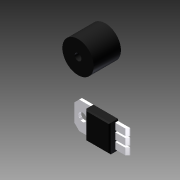
# Autodesk Inventor part: Breadboard
Saved by Autodesk Inventor 2012 (Build 160160000, 160)
## iProperties
Created: 2012-03-02
Part Number: Breadboard
Material: Default
Document SubType Name: Modeling
Designer: Lauszus
Density: 1 g/cm^3
Author: Lauszus
Autodesk Inventor part; units mm, degrees
ref_plane "YZ Plane" through (0, 0, 0) normal (1, 0, 0) x (0, 1, 0)
ref_plane "XZ Plane" through (0, 0, 0) normal (0, 1, 0) x (-1, 0, 0)
ref_plane "XY Plane" through (0, 0, 0) normal (0, 0, 1) x (1, 0, 0)
sketch "Sketch1" plane through (0, 0, 0) normal (0, 0, 1) x (1, 0, 0)
  line L0 (35.093, -7.2202) -> (-19.907, -7.2202)
  line L1 (-19.907, -7.2202) -> (-19.907, 74.7798)
  line L2 (-19.907, 74.7798) -> (35.093, 74.7798)
  line L3 (35.093, 74.7798) -> (35.093, -7.2202)
  line L4 (-1.6316, 73.7798) -> (15.8684, 73.7798)
  line L5 (15.8684, 73.7798) -> (15.8684, 38.2798)
  line L6 (15.8684, 38.2798) -> (-1.6316, 38.2798)
  line L7 (-1.6316, 38.2798) -> (-1.6316, 73.7798)
  circle A0 centre (7.5885, 28.2798) radius 5.75
  line L8 (12.233, 6.0025) -> (3.233, 6.0025)
  line L9 (3.233, 6.0025) -> (3.233, -3.9975)
  line L10 (3.233, -3.9975) -> (12.233, -3.9975)
  line L11 (12.233, -3.9975) -> (12.233, 6.0025)
  circle A1 centre (7.5885, 28.2798) radius 1.25
  line L12 (3.233, 6.0025) -> (-2.767, 6.0025)
  line L13 (-2.767, 6.0025) -> (-2.767, -3.9975)
  line L14 (-2.767, -3.9975) -> (3.233, -3.9975)
  line L15 (3.233, -3.9975) -> (3.233, 6.0025)
  line L16 (12.233, 5.3167) -> (16.7288, 5.3167)
  line L17 (16.7288, 5.3167) -> (16.7288, 2.7767)
  line L18 (16.7288, 2.7767) -> (12.233, 2.7767)
  line L19 (12.233, 2.7767) -> (12.233, 5.3167)
  line L20 (12.233, -1.5375) -> (12.233, 1.0025)
  line L21 (12.233, -3.4895) -> (12.233, -0.9495)
  line L22 (12.233, 2.2687) -> (16.7288, 2.2687)
  line L23 (16.7288, 2.2687) -> (16.7288, -0.2713)
  line L24 (16.7288, -0.2713) -> (12.233, -0.2713)
  line L25 (12.233, -0.2713) -> (12.233, 2.2687)
  line L26 (12.233, -0.7793) -> (16.7288, -0.7793)
  line L27 (16.7288, -0.7793) -> (16.7288, -3.3193)
  line L28 (16.7288, -3.3193) -> (12.233, -3.3193)
  line L29 (12.233, -3.3193) -> (12.233, -0.7793)
  circle A2 centre (0.233, 0.9987) radius 1.5
  circle A3 centre (0.3684, 66.2798) radius 0.75
  circle A4 centre (0.3684, 63.7398) radius 0.75
  circle A5 centre (0.3684, 61.1998) radius 0.75
  circle A6 centre (0.3684, 58.6598) radius 0.75
  circle A7 centre (0.3684, 56.1198) radius 0.75
  circle A8 centre (0.3684, 53.5798) radius 0.75
  circle A9 centre (0.3684, 51.0398) radius 0.75
  circle A10 centre (0.3684, 48.4998) radius 0.75
  circle A11 centre (13.8684, 66.2798) radius 0.75
  circle A12 centre (13.8684, 63.7398) radius 0.75
  circle A13 centre (13.8684, 61.1998) radius 0.75
  circle A14 centre (13.8684, 58.6598) radius 0.75
  circle A15 centre (13.8684, 56.1198) radius 0.75
  circle A16 centre (13.8684, 53.5798) radius 0.75
  circle A17 centre (13.8684, 51.0398) radius 0.75
  circle A18 centre (13.8684, 48.4998) radius 0.75
  line L30 (-17.907, 69.7798) -> (-16.407, 69.7798)
  line L31 (-16.407, 69.7798) -> (-16.407, -2.2202)
  line L32 (-16.407, -2.2202) -> (-17.907, -2.2202)
  line L33 (-17.907, -2.2202) -> (-17.907, 69.7798)
  line L34 (-15.367, -2.2202) -> (-13.867, -2.2202)
  line L35 (-13.867, -2.2202) -> (-13.867, 69.7798)
  line L36 (-13.867, 69.7798) -> (-15.367, 69.7798)
  line L37 (-15.367, 69.7798) -> (-15.367, -2.2202)
  line L38 (31.593, 69.7798) -> (33.093, 69.7798)
  line L39 (33.093, 69.7798) -> (33.093, -2.2202)
  line L40 (33.093, -2.2202) -> (31.593, -2.2202)
  line L41 (31.593, -2.2202) -> (31.593, 69.7798)
  line L42 (30.553, -2.2202) -> (29.053, -2.2202)
  line L43 (29.053, -2.2202) -> (29.053, 69.7798)
  line L44 (29.053, 69.7798) -> (30.553, 69.7798)
  line L45 (30.553, 69.7798) -> (30.553, -2.2202)
  line L46 (5.8684, 68.7798) -> (10.8684, 68.7798)
  line L47 (10.8684, 68.7798) -> (10.8684, 63.7798)
  line L48 (10.8684, 63.7798) -> (5.8684, 63.7798)
  line L49 (5.8684, 63.7798) -> (5.8684, 68.7798)
  line L50 (6.8684, 55.8198) -> (10.8684, 55.8198)
  line L51 (10.8684, 55.8198) -> (10.8684, 53.2798)
  line L52 (10.8684, 53.2798) -> (6.8684, 53.2798)
  line L53 (6.8684, 53.2798) -> (6.8684, 55.8198)
  line L54 (5.8684, 48.2798) -> (10.8684, 48.2798)
  line L55 (10.8684, 48.2798) -> (10.8684, 43.2798)
  line L56 (10.8684, 43.2798) -> (5.8684, 43.2798)
  line L57 (5.8684, 43.2798) -> (5.8684, 48.2798)
  circle A19 centre (0.8684, 71.2798) radius 1.5
  circle A20 centre (0.8684, 40.7798) radius 1.5
  point P0 (0, 0)
  dimension "d0" = 82
  dimension "d1" = 55
  dimension "d2" = 17.5
  dimension "d3" = 35.5
  dimension "d4" = 11.5
  dimension "d5" = 2.5
  dimension "d6" = 1
  dimension "d7" = 10
  dimension "d8" = 27.4955
  dimension "d9" = 9
  dimension "d10" = 10
  dimension "d16" = 6
  dimension "d17" = 22.86
  dimension "d18" = 19.2246
  dimension "d19" = 2.54
  dimension "d22" = 0.6858
  dimension "d24" = 10
  dimension "d25" = 2.54
  dimension "d26" = 0.508
  dimension "d27" = 4.4958
  dimension "d28" = 4.4958
  dimension "d29" = 2.54
  dimension "d30" = 4.4958
  dimension "d31" = 0.508
  dimension "d42" = 3
  dimension "d56" = 1.5
  dimension "d57" = 7.5
  dimension "d58" = 2
  dimension "d59" = 1.5
  dimension "d60" = 1.5
  dimension "d61" = 1.5
  dimension "d62" = 1.5
  dimension "d63" = 1.5
  dimension "d64" = 1.5
  dimension "d65" = 1.5
  dimension "d66" = 2.54
  dimension "d67" = 2.54
  dimension "d68" = 2.54
  dimension "d69" = 2.54
  dimension "d70" = 2.54
  dimension "d71" = 2.54
  dimension "d72" = 2.54
  dimension "d73" = 1.5
  dimension "d74" = 1.5
  dimension "d75" = 1.5
  dimension "d76" = 1.5
  dimension "d77" = 1.5
  dimension "d78" = 1.5
  dimension "d79" = 1.5
  dimension "d80" = 1.5
  dimension "d81" = 2.54
  dimension "d82" = 2.54
  dimension "d83" = 2.54
  dimension "d84" = 2.54
  dimension "d85" = 2.54
  dimension "d86" = 2.54
  dimension "d87" = 2.54
  dimension "d88" = 2
  dimension "d89" = 7.5
  dimension "d90" = 2
  dimension "d91" = 2
  dimension "d92" = 2
  dimension "d93" = 2
  dimension "d94" = 2
  constraints: 116 end point, 28 parallel, 21 centre point, 14 horizontal, 14 perpendicular, 4 point on line, 1 coincident, 1 midpoint
  measures "d0" distance of L0.end L1.end
  measures "d1" distance of L1.end L2.end
  measures "d2" distance of L4.start L4.end
  measures "d3" distance of L4.end L5.end
  measures "d4" diameter of A0
  measures "d5" diameter of A1
  measures "d6" distance between parallel lines of L2 L4
  measures "d7" distance from line of A0.centre L6
  measures "d8" distance from line of L1 A0.centre
  measures "d9" distance between parallel lines of L9 L11
  measures "d10" distance of L10.end L8.start
  measures "d16" distance of L8.end L12.end
  measures "d17" distance between parallel lines of L3 L11
  measures "d18" distance between parallel lines of L3 L5
  measures "d19" distance of L16.end L17.end
  measures "d22" distance between parallel lines of L8 L16
  measures "d24" distance of L14.end L8.end
  measures "d25" distance of L22.end L23.end
  measures "d26" distance between parallel lines of L18 L22
  measures "d27" distance of L16.start L16.end
  measures "d28" distance of L22.start L22.end
  measures "d29" distance of L26.end L27.end
  measures "d30" distance of L26.start L26.end
  measures "d31" distance between parallel lines of L24 L26
  measures "d42" diameter of A2
  measures "d56" diameter of A3
  measures "d57" distance from line of L4 A3.centre
  measures "d58" distance from line of L7 A3.centre
  measures "d59" diameter of A4
  measures "d60" diameter of A5
  measures "d61" diameter of A6
  measures "d62" diameter of A7
  measures "d63" diameter of A8
  measures "d64" diameter of A9
  measures "d65" diameter of A10
  measures "d66" distance of A4.centre A3.centre
  measures "d67" distance between centres of A5 A4
  measures "d68" distance between centres of A6 A5
  measures "d69" distance of A7.centre A6.centre
  measures "d70" distance between centres of A8 A7
  measures "d71" distance between centres of A9 A8
  measures "d72" distance between centres of A10 A9
  measures "d73" diameter of A11
  measures "d74" diameter of A12
  measures "d75" diameter of A13
  measures "d76" diameter of A14
  measures "d77" diameter of A15
  measures "d78" diameter of A16
  measures "d79" diameter of A17
  measures "d80" diameter of A18
  measures "d81" distance of A12.centre A11.centre
  measures "d82" distance between centres of A13 A12
  measures "d83" distance between centres of A14 A13
  measures "d84" distance of A15.centre A14.centre
  measures "d85" distance between centres of A16 A15
  measures "d86" distance between centres of A17 A16
  measures "d87" distance between centres of A18 A17
  measures "d88" distance from line of L5 A11.centre
  measures "d89" distance from line of L4 A11.centre
  measures "d90" distance from line of L5 A12.centre
  measures "d91" distance from line of L5 A13.centre
  measures "d92" distance from line of L5 A14.centre
  measures "d93" distance from line of L5 A15.centre
  measures "d94" distance from line of L5 A16.centre
extrude "Extrusion1" add sketch "Sketch1" along normal blind 3 draft -0.001 contours L11 L10 L9 L8
chamfer "Chamfer1" distance 0.381 angle 45 5 edges at (7.733, 6.0025, 3) (12.2329, 5.6596, 3) (12.2329, -2.4735, 3) (7.733, -3.9974, 3) (3.233, 1.0025, 3)
extrude "Extrusion2" add sketch "Sketch1" along normal blind 1 contours L9 L14 L13 L12 | A2
chamfer "Chamfer2" distance 1.778 angle 45 2 edges at (-2.767, -3.9975, 0.5) (-2.767, 6.0025, 0.5)
extrude "Extrusion3" cut sketch "Sketch1" along normal through all contours A2
extrude "Extrusion4" add sketch "Sketch1" along normal blind 1 contours L16 L17 L18 L11 | L22 L23 L24 L11 | L11 L26 L27 L28
chamfer "Chamfer3" distance 0.889 angle 45 3 edges at (16.7288, -2.0493, 1) (16.7288, 0.9987, 1) (16.7288, 4.0467, 1)
fillet "Fillet1" radius 0.127 9 edges at (14.0364, -3.3193, 1) (15.8398, -2.0493, 1) (14.0364, -0.7793, 1) (15.8398, 0.9987, 1) (14.0364, -0.2713, 1) (14.0364, 2.2687, 1) (14.0364, 2.7767, 1) (15.8398, 4.0467, 1) (14.0364, 5.3167, 1)
fillet "Fillet2" radius 0.127 3 edges at (16.7288, -2.0493, 0.111) (16.7288, 0.9987, 0.111) (16.7288, 4.0467, 0.111)
extrude "Extrusion5" add sketch "Sketch1" along normal blind 5 contours A1
extrude "Extrusion6" add sketch "Sketch1" along normal blind 10 contours A0
body "Solid1"
